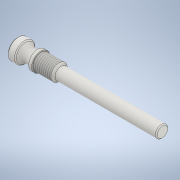
# Autodesk Inventor part: 轴
Saved by Autodesk Inventor 2020 (Build 240168000, 168)
## iProperties
CustomPartVersion: 1
Created: 2021-06-16
Part Number: 轴
Material: Steel
Document SubType Name: Modeling
Designer: dell
Density: 1 g/cm^3
Appearance: Steel
Length: 143.000 mm
Author: dell
Autodesk Inventor part; units mm, degrees
ref_plane "XZ Plane" through (0, 0, 0) normal (0, 1, 0) x (-1, 0, 0)
ref_plane "XY Plane" through (0, 0, 0) normal (0, 0, 1) x (1, 0, 0)
ref_plane "起始平面" through (0, 0, 0) normal (1, 0, 0) x (0, 1, 0)
sketch "主草图" plane through (0, 0, 0) normal (0, 0, 1) x (1, 0, 0)
  line L0 (0, 0) -> (143, 0)
  line L1 (0, 0) -> (0, 10)
  line L2 (8, 10) -> (8, 9)
  line L3 (0, 10) -> (8, 10)
  line L4 (23, 9) -> (23, 8)
  line L5 (8, 9) -> (23, 9)
  line L6 (43, 8) -> (43, 6)
  line L7 (23, 8) -> (43, 8)
  line L8 (143, 6) -> (143, 0)
  line L9 (43, 6) -> (143, 6)
  dimension "d3" = 20
  dimension "d4" = 18
  dimension "d5" = 16
  dimension "d6" = 12
  constraints: 20 end point, 5 vertical, 2 horizontal
  measures "d3" diameter of L3 L0
  measures "d4" diameter of L5 L0
  measures "d5" diameter of L7 L0
  measures "d6" diameter of L9 L0
revolve "旋转1" add sketch "主草图" angle 360 about axis through (0, 0, 0) along (1, 0, 0)
chamfer "倒角1" distance 1 angle 45 3 edges at (0, -10, 0) (8, -10, 0) (143, -6, 0)
fillet "圆角1" [suppressed]
chamfer "倒角2" distance 2 angle 45 1 edges at (43, -8, 0)
thread "螺纹1" size "M16x2" designation "M16" class "6g" standard "GB Metric profile" full length
sketch "草图3" plane through (0, 0, 0) normal (0, 1, 0) x (-1, 0, 0)
  line L0 (-23, -9) -> (-23, 9) construction
  line L1 (-8, -9) -> (-8, 9) construction
  line L2 (-23, 9) -> (-8, 9) construction
  line L3 (-20, 9) -> (-20, -9) construction
  line L4 (-23, -9) -> (-8, -9) construction
  arc A0 (-20, 9) -> (-8, 9) centre (-14, 14.2915) ccw
  line L5 (-20, 9) -> (-8, 9)
  line L6 (28.6, 0) -> (-171.6, 0) projected
  point P0 (0, 0)
  dimension "d17" = 3
  dimension "d18" = 8
  constraints: 4 end point, 2 point on circle, 2 point on line, 1 centre point, 1 vertical
  measures "d17" distance between parallel lines of L0 L3
  measures "d18" radius of A0
revolve "旋转2" cut sketch "草图3" angle 360 about axis through (-10, 0, 0) along (1, 0, 0)
equation "\"Length\" = 143"
